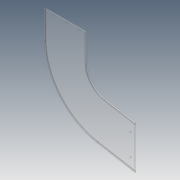
# Autodesk Inventor part: GE-12070-01
Saved by Autodesk Inventor 2012 (Build 160160000, 160)
## iProperties
Created: 2011-09-22
Part Number: GE-12070-01
Document SubType Name: Modeling
Designer: dfoster
Density: 1 g/cm^3
Description: Side
Material: Default
Title: Side
Author: dfoster
Autodesk Inventor part; units mm, degrees
ref_plane "YZ Plane" through (0, 0, 0) normal (1, 0, 0) x (0, 1, 0)
ref_plane "XZ Plane" through (0, 0, 0) normal (0, 1, 0) x (-1, 0, 0)
ref_plane "XY Plane" through (0, 0, 0) normal (0, 0, 1) x (1, 0, 0)
sketch "Sketch1" plane through (0, 0, 0) normal (0, 0, 1) x (1, 0, 0)
  line L0 (0, 0) -> (0, -161.1088)
  line L1 (0, 0) -> (244.475, 0)
  line L2 (244.475, 0) -> (244.475, -161.1088)
  line L3 (349.4217, -286.1793) -> (527.05, -317.5)
  line L4 (527.05, -317.5) -> (527.05, -565.7464)
  line L5 (527.05, -565.7464) -> (306.969, -526.9402)
  arc A0 (244.475, -161.1088) -> (349.4217, -286.1793) centre (371.475, -161.1088) ccw
  arc A1 (0, -161.1088) -> (306.969, -526.9402) centre (371.475, -161.1088) ccw
  dimension "d0" = 244.475
  dimension "d1" = 244.475
  dimension "d2" = 100
  dimension "d3" = 127
  dimension "d4" = 371.475
  dimension "d5" = 317.5
  dimension "d6" = 527.05
  constraints: 12 end point, 4 point on circle, 4 tangent, 2 centre point, 2 parallel, 2 perpendicular, 1 vertical
  measures "d0" distance of L0.start L1.end
  measures "d1" distance between parallel lines of L5 L3
  measures "d2" angle of L5 L0
  measures "d3" radius of A0
  measures "d4" radius of A1
  measures "d5" distance from line of L3.end L1
  measures "d6" distance between parallel lines of L4 L0
extrude "Extrusion1" add sketch "Sketch1" along normal blind 6.35
sketch "Sketch2" plane through (0, 0, 6.35) normal (0, 0, 1) x (1, 0, 0)
  line L0 (0, 0) -> (244.475, 0) projected
  line L1 (0, -161.1088) -> (0, 0) projected
  arc A0 (0, -161.1088) -> (306.969, -526.9402) centre (371.475, -161.1088) ccw projected
  line L2 (527.05, -565.7464) -> (306.969, -526.9402) projected
  line L3 (527.05, -317.5) -> (527.05, -565.7464) projected
  line L4 (349.4217, -286.1793) -> (527.05, -317.5) projected
  arc A1 (244.475, -161.1088) -> (349.4217, -286.1793) centre (371.475, -161.1088) ccw projected
  line L5 (244.475, 0) -> (244.475, -161.1088) projected
  arc A2 (239.7125, -161.1088) -> (348.5947, -290.8695) centre (371.475, -161.1088) ccw
  line L6 (348.5947, -290.8695) -> (527.05, -322.336)
  line L7 (527.05, -560.9105) -> (307.796, -522.2501)
  arc A3 (4.7625, -161.1088) -> (307.796, -522.2501) centre (371.475, -161.1088) ccw
  line L8 (4.7625, -161.1088) -> (4.7625, 0)
  line L9 (239.7125, 0) -> (239.7125, -161.1088)
  line L10 (7.9375, 0) -> (7.9375, -161.1088)
  arc A4 (7.9375, -161.1088) -> (308.3474, -519.1233) centre (371.475, -161.1088) ccw
  line L11 (308.3474, -519.1233) -> (527.05, -557.6865)
  line L12 (236.5375, 0) -> (236.5375, -161.1088)
  arc A5 (236.5375, -161.1088) -> (348.0433, -293.9962) centre (371.475, -161.1088) ccw
  line L13 (348.0433, -293.9962) -> (527.05, -325.5599)
  line L14 (4.7625, 0) -> (7.9375, 0)
  line L15 (239.7125, 0) -> (236.5375, 0)
  line L16 (527.05, -322.336) -> (527.05, -325.5599)
  line L17 (527.05, -560.9105) -> (527.05, -557.6865)
  dimension "d9" = 4.7625
  dimension "d10" = 4.7625
  dimension "d11" = 4.7625
  dimension "d12" = 4.7625
  dimension "d13" = 4.7625
  dimension "d14" = 4.7625
  dimension "d15" = 3.175
  dimension "d16" = 3.175
  dimension "d17" = 3.175
  dimension "d18" = 3.175
  constraints: 24 end point, 8 point on circle, 4 centre point, 4 point on line, 2 vertical, 1 collinear, 1 perpendicular, 2 other
  measures "d9" distance between parallel lines of L5 L9
  measures "d10" distance between parallel lines of L1 L8
  measures "d11" radial gap between concentric circles of A0 A3
  measures "d12" distance between parallel lines of L2 L7
  measures "d13" distance between parallel lines of L6 L4
  measures "d14" radial gap between concentric circles of A2 A1
  measures "d15" distance between parallel lines of L10 L8
  measures "d16" distance between parallel lines of L9 L12
  measures "d17" distance between parallel lines of L6 L13
  measures "d18" distance between parallel lines of L11 L7
extrude "Extrusion2" cut sketch "Sketch2" against normal blind 3.175 contours L0 L10 A4 L11 L3 L7 A3 L8 | L0 L9 A2 L6 L3 L13 A5 L12
hole "Hole1" at (496.8748, -377.825, 6.35) direction (0, 0, -1) diameter 6.731 depth 25.4 tip angle 118
pattern_linear "Rectangular Pattern1" count 2 spacing 127 along (0, -1, 0) of "Hole1"
hole "Hole2" at (200.025, -12.7, 6.35) direction (0, 0, -1) diameter 6.731 depth 25.4 tip angle 118
pattern_linear "Rectangular Pattern2" count 3 spacing 76.2 along (-1, 0, 0) of "Hole2"
equation "\"d1\" = d0"
equation "\"d4\" = d3 + d0"
equation "\"d9\" = d10"
equation "\"d11\" = d10"
equation "\"d12\" = d10"
equation "\"d13\" = d10"
equation "\"d14\" = d10"
body "Solid1"
